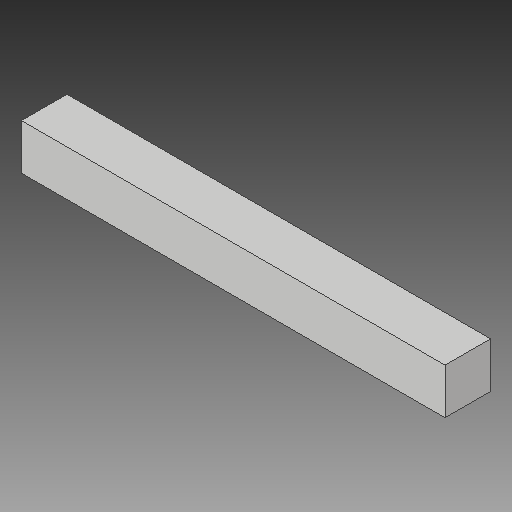
# Autodesk Inventor part: Top Frame
Saved by Autodesk Inventor 2018.1 (Build 221171000, 171)
## iProperties
Created: 2024-06-06
Part Number: Top Frame
Material: Generic
Document SubType Name: Modeling
Designer: Enrico
Density: 1 g/cm^3
Appearance: Default
Author: Enrico
Autodesk Inventor part; units mm, degrees
ref_plane "YZ Plane" through (0, 0, 0) normal (1, 0, 0) x (0, 1, 0)
ref_plane "XZ Plane" through (0, 0, 0) normal (0, 1, 0) x (-1, 0, 0)
ref_plane "XY Plane" through (0, 0, 0) normal (0, 0, 1) x (1, 0, 0)
ref_plane "Work Plane1" through (730.8614, 657.7874, 0.1) normal (0, 0, 1) x (1, 0, 0)
sketch "Sketch1" plane through (730.8614, 657.7874, 0.1) normal (0, 0, 1) x (1, 0, 0)
  line L0 (-25.6, -11.5) -> (-25.6, 11.5) construction
  line L1 (265.6, 11.5) -> (265.6, -11.5) construction
  line L2 (265.6, 0) -> (-25.6, 0) construction
  line L3 (305.9, 20) -> (-65.9, 20)
  line L4 (-65.9, 20) -> (-65.9, -20)
  line L5 (-65.9, -20) -> (305.9, -20)
  line L6 (305.9, -20) -> (305.9, 20)
  point P0 (-730.8614, -657.7874)
  dimension "d0" = 40
  dimension "d1" = 40.3
  dimension "d2" = 40.3
  constraints: 10 end point, 2 midpoint, 2 parallel, 1 horizontal, 1 perpendicular, 1 other
  measures "d0" distance between parallel lines of L5 L3
  measures "d1" distance between parallel lines of L6 L1
  measures "d2" distance between parallel lines of L0 L4
extrude "Extrusion1" add sketch "Sketch1" along normal blind 40
body "Solid1"
